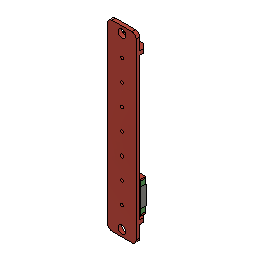
Linear Slide and Mount (Autodesk Fusion 360 design; units mm, degrees)
Autodesk Fusion 360 part; units mm, degrees
note: some values were not read from the file. Chosen so that the rebuilt part matches the saved one: how an offset face is resized. Set by a fixed rule: which sketch regions a step uses.
sketch "Sketch1" plane through (0, 0, 0) normal (0, 1, 0) x (1, 0, 0)
  line L0 (0, 0) -> (7, 0)
  line L1 (7, 0) -> (7, -5)
  line L2 (7, -5) -> (0, -5)
  line L3 (0, -5) -> (0, 0)
  line L4 (0, -1.5) -> (1, -1.5)
  line L5 (1, -1.5) -> (1, -2.25)
  line L6 (1, -2.25) -> (0, -2.25)
  line L7 (0, -2.25) -> (0, -1.5)
  line L8 (7, -1.5) -> (6, -1.5)
  line L9 (6, -1.5) -> (6, -2.25)
  line L10 (6, -2.25) -> (7, -2.25)
  line L11 (7, -2.25) -> (7, -1.5)
  dimension "d1" = 5
  dimension "d2" = 7
  dimension "d3" = 0.75
  dimension "d4" = 2.75
  dimension "d5" = 1
  measures "d3" distance of L4 L6
  measures "d4" distance of L2 L6
extrude "Extrude1" add sketch "Sketch1" along normal blind 100 contours L0 L1 L2 L3 L4 L5 L6 L8 L9 L10 makes body 1
chamfer "Chamfer2" distance 0.25 angle 45 24 edges at (3.5, 100, 0) (0, 100, 0.75) (0.5, 100, 1.5) (1, 100, 1.875) (0.5, 100, 2.25) (0, 100, 3.625) (3.5, 100, 5) (7, 100, 3.625) (6.5, 100, 2.25) (6, 100, 1.875) (6.5, 100, 1.5) (7, 100, 0.75) (3.5, 0, 0) (7, 0, 0.75) (6.5, 0, 1.5) (6, 0, 1.875) (6.5, 0, 2.25) (7, 0, 3.625) (3.5, 0, 5) (0, 0, 3.625) (0.5, 0, 2.25) (1, 0, 1.875) (0.5, 0, 1.5) (0, 0, 0.75) on bodies 1
chamfer "Chamfer1" distance 0.375 angle 45 8 edges at (0, 50, 0) (0, 50, 1.5) (0, 50, 2.25) (0, 50, 5) (7, 50, 2.25) (7, 50, 1.5) (7, 50, 0) (7, 50, 5) on bodies 1
sketch "Sketch2" plane through (0, 0, 0) normal (0, 0, -1) x (-1, 0, 0)
  line L0 (-6.625, 99.75) -> (-6.625, 0.25)
  line L1 (-6.625, 0.25) -> (-0.375, 0.25)
  line L2 (-0.375, 0.25) -> (-0.375, 99.75)
  line L3 (-0.375, 99.75) -> (-6.625, 99.75)
  circle A0 centre (-3.5, 5) radius 2
  line L4 (-6.75, 0) -> (-0.25, 0)
  line L5 (-3.5, 0) -> (-3.5, 5) construction
  circle A1 centre (-3.5, 20) radius 2
  circle A2 centre (-3.5, 35) radius 2
  circle A3 centre (-3.5, 50) radius 2
  circle A4 centre (-3.5, 65) radius 2
  circle A5 centre (-3.5, 80) radius 2
  circle A6 centre (-3.5, 95) radius 2
  dimension "d10" = 4
  dimension "d11" = 5
  dimension "d14" = 0
  dimension "d15" = 90
  measures "d10" diameter of A0
extrude "Extrude2" cut sketch "Sketch2" against normal blind 3 contours A0 | A1 | A2 | A3 | A4 | A5 | A6 bodies 1
sketch "Sketch3" plane through (0, 0, 0) normal (0, 0, -1) x (-1, 0, 0)
  circle A0 centre (-3.5, 35) radius 2
  circle A1 centre (-3.5, 95) radius 2
  circle A2 centre (-3.5, 50) radius 2
  circle A3 centre (-3.5, 20) radius 2
  circle A4 centre (-3.5, 80) radius 2
  circle A5 centre (-3.5, 65) radius 2
  circle A6 centre (-3.5, 5) radius 2
  line L0 (-6.625, 99.75) -> (-6.625, 0.25)
  line L1 (-6.625, 0.25) -> (-0.375, 0.25)
  line L2 (-0.375, 0.25) -> (-0.375, 99.75)
  line L3 (-0.375, 99.75) -> (-6.625, 99.75)
  line L4 (-6.625, 0.25) -> (-6.625, 99.75)
  line L5 (-6.625, 99.75) -> (-0.375, 99.75)
  line L6 (-0.375, 99.75) -> (-0.375, 0.25)
  line L7 (-0.375, 0.25) -> (-6.625, 0.25)
  circle A7 centre (-3.5, 5) radius 2
  circle A8 centre (-3.5, 20) radius 2
  circle A9 centre (-3.5, 35) radius 2
  circle A10 centre (-3.5, 50) radius 2
  circle A11 centre (-3.5, 65) radius 2
  circle A12 centre (-3.5, 80) radius 2
  circle A13 centre (-3.5, 95) radius 2
  circle A14 centre (-3.5, 95) radius 1.25
  circle A15 centre (-3.5, 80) radius 1.25
  circle A16 centre (-3.5, 65) radius 1.25
  circle A17 centre (-3.5, 50) radius 1.25
  circle A18 centre (-3.5, 35) radius 1.25
  circle A19 centre (-3.5, 20) radius 1.25
  circle A20 centre (-3.5, 5) radius 1.25
  dimension "d18" = 2.5
  measures "d18" diameter of A20
extrude "Extrude3" cut sketch "Sketch3" against normal blind 5 contours A14 | A15 | A16 | A17 | A18 | A19 | A20 bodies 1
sketch "Sketch4" plane through (0, 0, 0) normal (0, -1, 0) x (1, 0, 0)
  line L0 (1.25, 1.25) -> (0.25, 1.25)
  line L1 (0.25, 1.25) -> (0.25, 0.25)
  line L2 (0.25, 0.25) -> (6.75, 0.25)
  line L3 (6.75, 0.25) -> (6.75, 1.25)
  line L4 (6.75, 1.25) -> (5.75, 1.25)
  line L5 (5.75, 1.25) -> (5.75, 2.5)
  line L6 (5.75, 2.5) -> (6.75, 2.5)
  line L7 (6.75, 2.5) -> (6.75, 4.75)
  line L8 (6.75, 4.75) -> (0.25, 4.75)
  line L9 (0.25, 4.75) -> (0.25, 2.5)
  line L10 (0.25, 2.5) -> (1.25, 2.5)
  line L11 (1.25, 2.5) -> (1.25, 1.25)
  line L12 (0.375, 0) -> (6.625, 0)
  line L13 (6.625, 5) -> (0.375, 5)
  line L14 (12, -1) -> (-5, -1)
  line L15 (-5, -1) -> (-5, 3.2478)
  line L16 (-5, 3.2478) -> (12, 3.2478)
  line L17 (12, 3.2478) -> (12, -1)
  line L18 (3.5, -1) -> (3.5, 0) construction
  line L19 (0.25, 4.75) -> (6.75, 4.75)
  line L20 (6.75, 4.75) -> (6.75, 2.5)
  line L21 (6.75, 2.5) -> (5.75, 2.5)
  line L22 (5.75, 2.5) -> (5.75, 1.25)
  line L23 (5.75, 1.25) -> (6.75, 1.25)
  line L24 (6.75, 1.25) -> (6.75, 0.25)
  line L25 (6.75, 0.25) -> (0.25, 0.25)
  line L26 (0.25, 0.25) -> (0.25, 1.25)
  line L27 (0.25, 1.25) -> (1.25, 1.25)
  line L28 (1.25, 1.25) -> (1.25, 2.5)
  line L29 (1.25, 2.5) -> (0.25, 2.5)
  line L30 (0.25, 2.5) -> (0.25, 4.75)
  line L31 (6.05, 2.2) -> (7.05, 2.2)
  line L32 (7.05, 2.2) -> (7.05, 5.05)
  line L33 (7.05, 5.05) -> (-0.05, 5.05)
  line L34 (-0.05, 5.05) -> (-0.05, 2.2)
  line L35 (-0.05, 2.2) -> (0.95, 2.2)
  line L36 (0.95, 2.2) -> (0.95, 1.55)
  line L37 (0.95, 1.55) -> (-0.05, 1.55)
  line L38 (-0.05, 1.55) -> (-0.05, -0.05)
  line L39 (-0.05, -0.05) -> (7.05, -0.05)
  line L40 (7.05, -0.05) -> (7.05, 1.55)
  line L41 (7.05, 1.55) -> (6.05, 1.55)
  line L42 (6.05, 1.55) -> (6.05, 2.2)
  circle A0 centre (3.5, -0.5) radius 0.25
  dimension "d21" = 1.7522
  dimension "d22" = 6
  dimension "d23" = 17
  dimension "d24" = 0.3
  dimension "d25" = 0.5
  measures "d21" distance of L13 L16
  measures "d22" distance of L13 L14
  measures "d24" distance of L6
  measures "d25" diameter of A0
extrude "Extrude4" add sketch "Sketch4" against normal blind 22.5 separate body contours L14 L15 L16 L17 L31 L32 L34 L35 L36 L37 L38 L39 L40 L41 L42 makes body 2
sketch "Sketch5" plane through (0, 0, 0) normal (0, -1, 0) x (1, 0, 0)
  circle A0 centre (3.5, -0.5) radius 0.25
  line L0 (6.05, 1.55) -> (7.05, 1.55)
  line L1 (7.05, 1.55) -> (7.05, -0.05)
  line L2 (7.05, -0.05) -> (-0.05, -0.05)
  line L3 (-0.05, -0.05) -> (-0.05, 1.55)
  line L4 (-0.05, 1.55) -> (0.95, 1.55)
  line L5 (0.95, 1.55) -> (0.95, 2.2)
  line L6 (0.95, 2.2) -> (-0.05, 2.2)
  line L7 (-0.05, 2.2) -> (-0.05, 3.2478)
  line L8 (-0.05, 3.2478) -> (-5, 3.2478)
  line L9 (-5, 3.2478) -> (-5, -1)
  line L10 (-5, -1) -> (12, -1)
  line L11 (12, -1) -> (12, 3.2478)
  line L12 (12, 3.2478) -> (7.05, 3.2478)
  line L13 (7.05, 3.2478) -> (7.05, 2.2)
  line L14 (7.05, 2.2) -> (6.05, 2.2)
  line L15 (6.05, 2.2) -> (6.05, 1.55)
  circle A1 centre (3.5, -0.5) radius 0.25
  line L16 (7.05, 1.55) -> (6.05, 1.55)
  line L17 (6.05, 1.55) -> (6.05, 2.2)
  line L18 (6.05, 2.2) -> (7.05, 2.2)
  line L19 (7.05, 2.2) -> (7.05, 3.2478)
  line L20 (7.05, 3.2478) -> (12, 3.2478)
  line L21 (12, 3.2478) -> (12, -1)
  line L22 (12, -1) -> (-5, -1)
  line L23 (-5, -1) -> (-5, 3.2478)
  line L24 (-5, 3.2478) -> (-0.05, 3.2478)
  line L25 (-0.05, 3.2478) -> (-0.05, 2.2)
  line L26 (-0.05, 2.2) -> (0.95, 2.2)
  line L27 (0.95, 2.2) -> (0.95, 1.55)
  line L28 (0.95, 1.55) -> (-0.05, 1.55)
  line L29 (-0.05, 1.55) -> (-0.05, -0.05)
  line L30 (-0.05, -0.05) -> (7.05, -0.05)
  line L31 (7.05, -0.05) -> (7.05, 1.55)
  line L32 (7.15, 2.1) -> (6.15, 2.1)
  line L33 (6.15, 2.1) -> (6.15, 1.65)
  line L34 (6.15, 1.65) -> (7.15, 1.65)
  line L35 (7.15, 1.65) -> (7.15, -0.15)
  line L36 (7.15, -0.15) -> (-0.15, -0.15)
  line L37 (-0.15, -0.15) -> (-0.15, 1.65)
  line L38 (-0.15, 1.65) -> (0.85, 1.65)
  line L39 (0.85, 1.65) -> (0.85, 2.1)
  line L40 (0.85, 2.1) -> (-0.15, 2.1)
  line L41 (-0.15, 2.1) -> (-0.15, 3.1478)
  line L42 (-0.15, 3.1478) -> (-4.9, 3.1478)
  line L43 (-4.9, 3.1478) -> (-4.9, -0.9)
  line L44 (-4.9, -0.9) -> (11.9, -0.9)
  line L45 (11.9, -0.9) -> (11.9, 3.1478)
  line L46 (11.9, 3.1478) -> (7.15, 3.1478)
  line L47 (7.15, 3.1478) -> (7.15, 2.1)
  line L48 (11.9, 3.1478) -> (11.9, 3.2478)
  line L49 (-4.9, 3.1478) -> (-4.9, 3.2478)
  dimension "d28" = 0.1
  measures "d28" distance of L14
  measures "d82" distance of L41
extrude "Extrude5" cut sketch "Sketch5" against normal blind 4.5 contours L8 L9 L10 L11 L12 L20 L21 L22 L23 L24 L43 L44 L45 L48 L49 bodies 2
sketch "Sketch6" plane through (0, 22.5, 0) normal (0, 1, 0) x (-1, 0, 0)
  circle A0 centre (-3.5, -0.5) radius 0.25
  line L0 (-7.05, 1.55) -> (-6.05, 1.55)
  line L1 (-6.05, 1.55) -> (-6.05, 2.2)
  line L2 (-6.05, 2.2) -> (-7.05, 2.2)
  line L3 (-7.05, 2.2) -> (-7.05, 3.2478)
  line L4 (-7.05, 3.2478) -> (-12, 3.2478)
  line L5 (-12, 3.2478) -> (-12, -1)
  line L6 (-12, -1) -> (5, -1)
  line L7 (5, -1) -> (5, 3.2478)
  line L8 (5, 3.2478) -> (0.05, 3.2478)
  line L9 (0.05, 3.2478) -> (0.05, 2.2)
  line L10 (0.05, 2.2) -> (-0.95, 2.2)
  line L11 (-0.95, 2.2) -> (-0.95, 1.55)
  line L12 (-0.95, 1.55) -> (0.05, 1.55)
  line L13 (0.05, 1.55) -> (0.05, -0.05)
  line L14 (0.05, -0.05) -> (-7.05, -0.05)
  line L15 (-7.05, -0.05) -> (-7.05, 1.55)
  line L16 (4.9, -0.9) -> (4.9, 3.2478)
  line L17 (4.9, 3.2478) -> (5, 3.2478)
  line L18 (5, 3.2478) -> (5, -1)
  line L19 (5, -1) -> (-12, -1)
  line L20 (-12, -1) -> (-12, 3.2478)
  line L21 (-12, 3.2478) -> (-11.9, 3.2478)
  line L22 (-11.9, 3.2478) -> (-11.9, -0.9)
  line L23 (-11.9, -0.9) -> (4.9, -0.9)
extrude "Extrude6" cut sketch "Sketch6" against normal blind 4.5 contours L4 L5 L6 L7 L8 L16 L17 L18 L19 L20 L21 L22 L23 bodies 2
chamfer "Chamfer3" distance 0.5 angle 45 8 edges at (11.9, 20.25, -0.9) (11.9, 20.25, 3.2478) (11.9, 2.25, -0.9) (11.9, 2.25, 3.2478) (-4.9, 20.25, -0.9) (-4.9, 20.25, 3.2478) (-4.9, 2.25, -0.9) (-4.9, 2.25, 3.2478) on bodies 2
sketch "Sketch7" plane through (0, 0, -1) normal (0, 0, -1) x (-1, 0, 0)
  line L0 (5, 18) -> (-12, 18)
  line L1 (-12, 18) -> (-12, 4.5)
  line L2 (-12, 4.5) -> (5, 4.5)
  line L3 (5, 4.5) -> (5, 18)
  line L4 (-3.5, 18) -> (-3.5, 4.5) construction
  line L5 (2.5, 15.25) -> (-9.5, 15.25) construction
  line L6 (-9.5, 15.25) -> (-9.5, 7.25) construction
  line L7 (-9.5, 7.25) -> (2.5, 7.25) construction
  line L8 (2.5, 7.25) -> (2.5, 15.25) construction
  line L9 (2.5, 15.25) -> (-9.5, 7.25) construction
  line L10 (-9.5, 15.25) -> (2.5, 7.25) construction
  circle A0 centre (-9.5, 15.25) radius 1
  circle A1 centre (-9.5, 7.25) radius 1
  circle A2 centre (2.5, 7.25) radius 1
  circle A3 centre (2.5, 15.25) radius 1
  dimension "d34" = 8
  dimension "d35" = 12
  dimension "d36" = 2
  measures "d36" diameter of A2
extrude "Extrude7" cut sketch "Sketch7" against normal blind 3.5 contours A0 | A1 | A2 | A3 bodies 2
thread "Thread1" "ISO Metric profile 2.0 M2x0.4 6H" major diameter 2.074 minor diameter 1.623 pitch 0.4 angle 60 resizes the face on face at (8.505, 7.1504, 1.3333) on bodies 2
thread "Thread2" "ISO Metric profile 2.0 M2x0.4 6H" major diameter 2.074 minor diameter 1.623 pitch 0.4 angle 60 resizes the face on face at (8.505, 15.1504, 1.3333) on bodies 2
thread "Thread3" "ISO Metric profile 2.0 M2x0.4 6H" major diameter 2.074 minor diameter 1.623 pitch 0.4 angle 60 resizes the face on face at (-3.495, 7.1504, 1.3333) on bodies 2
thread "Thread4" "ISO Metric profile 2.0 M2x0.4 6H" major diameter 2.074 minor diameter 1.623 pitch 0.4 angle 60 resizes the face on face at (-3.495, 15.1504, 1.3333) on bodies 2
sketch "Sketch8" plane through (0, 0, -1) normal (0, 0, -1) x (-1, 0, 0)
  circle A0 centre (-9.5, 7.25) radius 0.8115
  circle A1 centre (2.5, 7.25) radius 0.8115
  circle A2 centre (-9.5, 15.25) radius 0.8115
  circle A3 centre (2.5, 15.25) radius 0.8115
  line L0 (5, 18) -> (-12, 18)
  line L1 (-12, 18) -> (-12, 4.5)
  line L2 (-12, 4.5) -> (5, 4.5)
  line L3 (5, 4.5) -> (5, 18)
  line L4 (-11.9, 22.5) -> (-11.9, 18)
  line L5 (4.9, 18) -> (4.9, 22.5)
  line L6 (4.9, 0) -> (4.9, 4.5)
  line L7 (-11.9, 4.5) -> (-11.9, 0)
  line L8 (-11.9, 21.5) -> (4.9, 21.5)
  line L9 (-11.9, 1) -> (4.9, 1)
  line L10 (-11.4, 22.5) -> (4.4, 22.5)
  line L11 (4.4, 0) -> (-11.4, 0)
  dimension "d39" = 1
  dimension "d40" = 1
  measures "d39" distance of L8 L10
  measures "d40" distance of L9 L11
split_face "SplitFace1" 16 faces at (-4.5667, 21, -0.7333) (-4.9, 21, 0.6493) (-4.7333, 21, 2.9144) (-1.5, 13.5, 3.2478) (6.1333, 21, -0.9) (11.5667, 21, -0.7333) (11.9, 21, 1.6985) (11.7333, 21, 2.9144) (8.5, 9, 3.2478) (11.7333, 1.5, -0.5667) (0.8667, 3, -0.9) (11.9, 3, 1.6985) (11.5667, 1.5, 3.0811) (-4.9, 3, 1.6985) (-4.5667, 1.5, -0.7333) (-4.7333, 1.5, 2.9144) by curves path "Sketch8" along L9 on bodies 2
split_face "SplitFace2" 9 faces at (6.1333, 21, -0.9) (11.5667, 21, -0.7333) (11.9, 21, 1.6985) (11.7333, 21, 2.9144) (8.5, 13.8333, 3.2478) (-4.5667, 21, -0.7333) (-4.9, 21, 0.6493) (-1.5, 13.8333, 3.2478) (-4.7333, 21, 2.9144) by curves path "Sketch8" along L8 on bodies 2
sketch "Sketch9" plane through (0, 0, 3.2478) normal (0, 0, 1) x (1, 0, 0)
  line L0 (11.4, 21.5) -> (7.05, 21.5)
  line L1 (7.05, 21.5) -> (7.05, 1)
  line L2 (7.05, 1) -> (11.4, 1)
  line L3 (11.4, 1) -> (11.4, 4.5)
  line L4 (11.4, 4.5) -> (12, 4.5)
  line L5 (12, 4.5) -> (12, 18)
  line L6 (12, 18) -> (11.4, 18)
  line L7 (11.4, 18) -> (11.4, 21.5)
  line L8 (-5, 18) -> (12, 18)
  line L9 (12, 18) -> (12, 4.5)
  line L10 (12, 4.5) -> (-5, 4.5)
  line L11 (-5, 4.5) -> (-5, 18)
split_face "SplitFace3" 2 faces at (8.5, 9, 3.2478) (-1.5, 13.5, 3.2478) by curves path "Sketch9" along L10 L11 L8 L9 on bodies 2
copy_body "Body->Comp1" bodies 1 removing the originals makes body 3 in component "Linear Slide"
copy_body "Body->Comp2" bodies 2 removing the originals makes body 4 in component "Carriage"
sketch "Sketch10" plane through (0, 0, 5) normal (0, 0, 1) x (1, 0, 0)
  circle A0 centre (3.5, 65) radius 1.25
  circle A1 centre (3.5, 5) radius 1.25
  circle A2 centre (3.5, 50) radius 1.25
  circle A3 centre (3.5, 80) radius 1.25
  circle A4 centre (3.5, 20) radius 1.25
  circle A5 centre (3.5, 35) radius 1.25
  circle A6 centre (3.5, 95) radius 1.25
  line L0 (6.625, 0.25) -> (6.625, 99.75)
  line L1 (6.625, 99.75) -> (0.375, 99.75)
  line L2 (0.375, 99.75) -> (0.375, 0.25)
  line L3 (0.375, 0.25) -> (6.625, 0.25)
  circle A7 centre (3.5, 35) radius 2
  circle A8 centre (3.5, 95) radius 2
  circle A9 centre (3.5, 50) radius 2
  circle A10 centre (3.5, 20) radius 2
  circle A11 centre (3.5, 80) radius 2
  circle A12 centre (3.5, 65) radius 2
  circle A13 centre (3.5, 5) radius 2
  line L4 (6.625, 99.75) -> (6.625, 0.25)
  line L5 (6.625, 0.25) -> (0.375, 0.25)
  line L6 (0.375, 0.25) -> (0.375, 99.75)
  line L7 (0.375, 99.75) -> (6.625, 99.75)
  line L8 (-6.5, 114.5) -> (13.5, 114.5)
  line L9 (13.5, 114.5) -> (13.5, -14.5)
  line L10 (13.5, -14.5) -> (-6.5, -14.5)
  line L11 (-6.5, -14.5) -> (-6.5, 114.5)
  line L12 (-0.225, -0.35) -> (7.225, -0.35)
  line L13 (7.225, -0.35) -> (7.225, 100.35)
  line L14 (7.225, 100.35) -> (-0.225, 100.35)
  line L15 (-0.225, 100.35) -> (-0.225, -0.35)
  line L16 (0.375, 50) -> (6.625, 50)
  line L17 (9.85, 107.15) -> (-2.85, 107.15)
  line L18 (-2.85, 107.15) -> (-2.85, -7.15)
  line L19 (-2.85, -7.15) -> (9.85, -7.15)
  line L20 (9.85, -7.15) -> (9.85, 107.15)
  line L21 (9.85, 107.15) -> (-2.85, -7.15) construction
  line L22 (-2.85, 107.15) -> (9.85, -7.15) construction
  line L23 (12.1614, 109.4614) -> (7.5386, 109.4614) construction
  line L24 (7.5386, 109.4614) -> (7.5386, 104.8386) construction
  line L25 (7.5386, 104.8386) -> (12.1614, 104.8386) construction
  line L26 (12.1614, 104.8386) -> (12.1614, 109.4614) construction
  line L27 (12.1614, 109.4614) -> (7.5386, 104.8386) construction
  line L28 (7.5386, 109.4614) -> (12.1614, 104.8386) construction
  line L29 (-6.5, 50) -> (13.5, 50) construction
  line L30 (-5.1614, 109.4614) -> (-5.1614, 104.8386) construction
  line L31 (-0.5386, 109.4614) -> (-5.1614, 109.4614) construction
  line L32 (-5.1614, 104.8386) -> (-0.5386, 104.8386) construction
  line L33 (-0.5386, 104.8386) -> (-0.5386, 109.4614) construction
  line L34 (7.5386, -4.8386) -> (7.5386, -9.4614) construction
  line L35 (12.1614, -4.8386) -> (7.5386, -4.8386) construction
  line L36 (7.5386, -9.4614) -> (12.1614, -9.4614) construction
  line L37 (12.1614, -9.4614) -> (12.1614, -4.8386) construction
  line L38 (-5.1614, -4.8386) -> (-5.1614, -9.4614) construction
  line L39 (-0.5386, -4.8386) -> (-5.1614, -4.8386) construction
  line L40 (-5.1614, -9.4614) -> (-0.5386, -9.4614) construction
  line L41 (-0.5386, -9.4614) -> (-0.5386, -4.8386) construction
  circle A14 centre (3.5, 95) radius 1
  circle A15 centre (3.5, 80) radius 1
  circle A16 centre (3.5, 65) radius 1
  circle A17 centre (3.5, 50) radius 1.25 construction
  circle A18 centre (3.5, 50) radius 1
  circle A19 centre (3.5, 35) radius 1
  circle A20 centre (3.5, 20) radius 1
  circle A21 centre (3.5, 5) radius 1
  line L42 (8.625, -1.75) -> (8.625, 101.75)
  line L43 (8.625, 101.75) -> (-1.625, 101.75)
  line L44 (-1.625, 101.75) -> (-1.625, -1.75)
  line L45 (-1.625, -1.75) -> (8.625, -1.75)
  line L46 (3.5, 114.5) -> (3.5, -14.5)
  circle A22 centre (3.5, -10) radius 2.75
  circle A23 centre (3.5, 110) radius 2.75
  dimension "d45" = 0.6
  dimension "d46" = 12.7
  dimension "d47" = 114.3
  dimension "d48" = 4.6228
  dimension "d49" = 4.6228
  dimension "d50" = 20
  dimension "d51" = 129
  dimension "d54" = -12.7
  dimension "d55" = -114.3
  dimension "d56" = 2
  dimension "d59" = 2
  dimension "d80" = 5.5
  dimension "d82" = 120
  dimension "d83" = 15
  measures "d45" distance of L3
  measures "d56" diameter of A14
  measures "d59" distance of L0
  measures "d80" diameter of A22
extrude "Extrude8" add sketch "Sketch10" along normal blind 2.54 separate body contours A0 A16 L46 | A0 A12 L46 | A0 A16 L46 | A0 A12 L46 | L0 L1 A8 A9 A11 A12 L4 L7 L16 L46 | L1 L2 A8 A9 A11 A12 L6 L7 L16 L46 | A3 A11 L46 | A3 A11 L46 | A2 A9 L16 L46 | A2 A9 L16 L46 | A3 A15 L46 | A3 A15 L46 | L0 L3 A7 A9 A10 A13 L4 L5 L16 L46 | A2 A9 L16 L46 | A2 A9 L16 L46 | L2 L3 A7 A9 A10 A13 L5 L6 L16 L46 | A2 L16 A18 L46 | A2 L16 A18 L46 | A6 A8 L46 | A6 A8 L46 | A2 L16 A18 L46 | L0 L1 L3 L4 L5 L7 L12 L13 L14 L46 | L1 L2 L3 L5 L6 L7 L12 L14 L15 L46 | A2 L16 A18 L46 | A6 A14 L46 | A6 A14 L46 | A5 A7 L46 | A5 A7 L46 | L12 L13 L14 L42 L43 L45 L46 | L12 L14 L15 L43 L44 L45 L46 | A4 A10 L46 | A4 A10 L46 | A1 A13 L46 | A1 A13 L46 | L17 L19 L20 L42 L43 L45 L46 | L17 L18 L19 L43 L44 L45 L46 | A4 A20 L46 | A4 A20 L46 | A1 A21 L46 | A1 A21 L46 | L8 L9 L10 L17 L19 L20 L46 A22 A23 | L8 L10 L11 L17 L18 L19 L46 A22 A23 makes body 5
extrude "Extrude10" add sketch "Sketch10" against normal blind 1 contours L12 L13 L14 L42 L43 L45 L46 | L12 L14 L15 L43 L44 L45 L46 bodies 5
sketch "Sketch12" plane through (0, 0, 5) normal (0, 0, 1) x (1, 0, 0)
  circle A0 centre (9.85, -7.15) radius 4.064
  line L0 (13.5, 0) -> (-6.5, 0)
  line L1 (-6.5, 0) -> (-6.5, -3.086)
  line L2 (-6.5, -3.086) -> (13.5, -3.086)
  line L3 (13.5, -3.086) -> (13.5, 0)
  line L4 (13.5, 114.5) -> (13.5, -14.5)
  line L5 (13.5, -14.5) -> (13.5, 114.5)
  line L6 (-6.5, -14.5) -> (-6.5, 114.5)
  line L7 (-6.5, 114.5) -> (-6.5, -14.5)
  line L8 (7.05, 0) -> (11.4, 0)
  circle A1 centre (9.85, 107.15) radius 4.064
  line L9 (0.25, 100) -> (6.75, 100)
  line L10 (13.5, 103.086) -> (-6.5, 103.086)
  line L11 (-6.5, 103.086) -> (-6.5, 100)
  line L12 (-6.5, 100) -> (13.5, 100)
  line L13 (13.5, 100) -> (13.5, 103.086)
  dimension "d67" = 8.128
  dimension "d70" = 8.128
  measures "d67" diameter of A0
  measures "d70" diameter of A1
extrude "Extrude9" add sketch "Sketch12" against normal blind 5.9 contours L0 L1 L2 L3 L4 L5 L6 L7 L8 | L4 L5 L6 L7 L9 L10 L11 L12 L13 bodies 5
move_face "OffsetFaces1" offset -0.3 2 faces at (4.7417, 0, 0.7333) (2.2583, 100, 0.7333) on bodies 5
chamfer "Chamfer4" distance 3 angle 45 4 edges at (13.5, -1.693, -0.9) (-6.5, -1.693, -0.9) (13.5, 101.693, -0.9) (-6.5, 101.693, -0.9) on bodies 5
fillet "Fillet1" radius 3 4 edges at (13.5, -14.5, 6.27) (-6.5, -14.5, 6.27) (13.5, 114.5, 6.27) (-6.5, 114.5, 6.27) on bodies 5
copy_body "Body->Comp3" bodies 5 removing the originals makes body 6 in component "Linear Slide Mount 1"
component "Linear Slide" placed x (1, 0, 0) y (0, 1, 0) z (0, 0, 1) at (0, 0, 0)
component "Carriage" placed x (1, 0, 0) y (0, 1, 0) z (0, 0, 1) at (0, 0, 0)
component "Linear Slide Mount 1" placed x (1, 0, 0) y (0, 1, 0) z (0, 0, 1) at (0, 0, 0)
equation "d82 = ( 15 * 8 ) * 1 mm"
